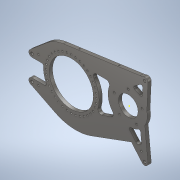
# Autodesk Inventor part: DTR-6
Saved by Autodesk Inventor 2021 (Build 250183000, 183)
## iProperties
Created: 2018-12-06
Part Number: DTR-6
Material: Aluminum 6061
Document SubType Name: Modeling
Designer: Lucas Foulk
Density: 2.7 g/cm^3
Appearance: Semi-Polished
Description: Right Mounting Plate
Material_Size: 1/2 Aluminum Plate
Quantity: 1
Author: Lucas Foulk
Autodesk Inventor part; units mm, degrees
ref_plane "YZ Plane" through (0, 0, 0) normal (1, 0, 0) x (0, 1, 0)
ref_plane "XZ Plane" through (0, 0, 0) normal (0, 1, 0) x (-1, 0, 0)
ref_plane "XY Plane" through (0, 0, 0) normal (0, 0, 1) x (1, 0, 0)
sketch "Sketch14" plane through (0, 0, 0) normal (0, 0, 1) x (1, 0, 0)
  circle A0 centre (0, 0) radius 69.85
  circle A1 centre (59.6616, 114.3) radius 12.7
  circle A2 centre (59.6616, -157.9372) radius 12.7
  circle A3 centre (-225.4026, -38.1) radius 107.95
  line L0 (52.1743, 124.5582) -> (-41.1802, 56.42)
  line L1 (72.3489, 113.732) -> (67.9766, 16.0689)
  line L2 (59.6616, 114.3) -> (0, 0)
  line L3 (0, 0) -> (59.6616, -157.9372)
  line L4 (72.2989, -156.6771) -> (60.2073, -35.4133)
  line L5 (50.0015, -166.1818) -> (-53.1301, -45.3456)
  line L6 (-547.6025, 1708.7209) -> (-492.7385, 1708.7209)
  circle A4 centre (-377.8026, -107.1372) radius 12.7
  circle A5 centre (-377.8026, -12.7) radius 12.7
  line L7 (-377.8026, -25.4) -> (-332.603, -25.4)
  line L8 (-377.8026, -94.4372) -> (-317.4859, -94.4372)
  line L9 (59.6616, 114.3) -> (59.6616, -157.9372)
  line L10 (-380.0803, -119.6313) -> (-244.7629, -144.2997)
  line L11 (-383.8817, -1.5494) -> (-277.0748, 56.6797)
  point P0 (49.5036, 49.279)
  point P1 (31.1227, 62.5332)
  point P2 (49.5036, 49.279)
  point P3 (-216.3804, 69.4723)
  point P4 (27.7497, 64.1013)
  point P5 (-222.5423, 69.8121)
  point P6 (64.0721, 27.817)
  point P7 (-119.2874, -57.9179)
  point P8 (35.0174, 60.4384)
  point P9 (30.2851, 62.9431)
  point P10 (30.2566, 62.9568)
  point P11 (-183.3373, 61.3169)
  point P12 (-197.0061, 66.0482)
  point P13 (-176.345, 58.059)
  dimension "d96" = 215.9
  dimension "d99" = 139.7
  dimension "d97" = 54.864
  dimension "d98" = 228.6
  dimension "d100" = 25.4
  dimension "d101" = 25.4
  dimension "d102" = 152.4
  dimension "d103" = 152.4
  dimension "d104" = 94.4372
  dimension "d105" = 25.4
  dimension "d108" = 272.2372
  dimension "d109" = 38.1
  dimension "d132" = 127
  dimension "d133" = 437.4642
  dimension "d207" = 25
  dimension "d208" = 15
  constraints: 24 end point, 8 point on circle, 8 tangent, 4 centre point, 3 horizontal, 2 coincident, 2 equal radius, 1 vertical, 30 other
  measures "d97" distance of L6.start L6.end
  measures "d98" distance of point (-225.403, -38.1) point (0, 0)
  measures "d100" diameter of A1
  measures "d101" diameter of A4
  measures "d102" horizontal distance of A4.centre point (-225.403, -38.1)
  measures "d103" horizontal distance of A5.centre point (-225.403, -38.1)
  measures "d104" distance of A4.centre A5.centre
  measures "d105" vertical distance of A5.centre point (-225.403, -38.1)
  measures "d108" distance of L9.start L9.end
  measures "d109" vertical distance of point (-225.403, -38.1) point (0, 0)
  measures "d132" vertical distance of L9.start A5.centre
  measures "d133" horizontal distance of L9.start A5.centre
  measures "d207" angle of L2 L1
  measures "d208" angle of L3 L4
extrude "Extrusion13" add sketch "Sketch14" along normal blind 12.7
sketch "Sketch15" plane through (0, 0, 12.7) normal (0, 0, 1) x (1, 0, 0)
  arc A0 (-383.8817, -1.5494) -> (-377.8026, -25.4) centre (-377.8026, -12.7) ccw projected
  arc A1 (-377.8026, -94.4372) -> (-380.0803, -119.6313) centre (-377.8026, -107.1372) ccw projected
  arc A2 (50.0015, -166.1818) -> (72.2989, -156.6771) centre (59.6616, -157.9372) ccw projected
  arc A3 (72.3489, 113.732) -> (52.1743, 124.5582) centre (59.6616, 114.3) ccw projected
  point P0 (0, 0)
  constraints: 4 coincident
hole "Hole4" at (-377.8026, -12.7, 12.7) at (-377.8026, -107.1372, 12.7) at (59.6616, -157.9372, 12.7) at (59.6616, 114.3, 12.7) direction (0, 0, -1) diameter 9.8044 depth 12.2936 tip angle 118 clearance for "Flat Head Machine Screw (82)" size "3/8" standard "Ansi Unified Screw Threads"
sketch "Sketch18" plane through (0, 0, 12.7) normal (0, 0, 1) x (1, 0, 0)
  arc A0 (-244.7629, -144.2997) -> (-277.0748, 56.6797) centre (-225.4026, -38.1) ccw projected
  arc A1 (-41.1802, 56.42) -> (-53.1301, -45.3456) centre (0, 0) ccw projected
  arc A2 (-36.2787, -59.6899) -> (-53.8815, 44.45) centre (0, 0) ccw
  line L0 (-189.9226, -140.0528) -> (22.9577, -65.9694)
  line L1 (-132.5746, -93.2013) -> (-36.2787, -59.6899)
  line L2 (-225.4026, 69.85) -> (0, 69.85)
  line L3 (-155.8419, 44.45) -> (-53.8815, 44.45)
  arc A3 (-155.8419, 44.45) -> (-225.4026, 69.85) centre (-225.4026, -38.1) ccw
  arc A4 (-189.9226, -140.0528) -> (-132.5746, -93.2013) centre (-225.4026, -38.1) ccw
  dimension "d134" = 25.4
  dimension "d135" = 25.4
  constraints: 11 point on circle, 8 end point, 4 tangent, 3 centre point, 2 coincident, 2 parallel, 1 concentric
  measures "d134" distance between parallel lines of L2 L3
  measures "d135" distance between parallel lines of L0 L1
extrude "Extrusion15" add sketch "Sketch18" against normal up to surface (12.7 mm away) contours A0 L1 A2 L0 | A0 L2 A2 A1 L3
sketch "Sketch21" plane through (0, 0, 12.7) normal (0, 0, 1) x (1, 0, 0)
  line L0 (-13.2861, -92.0295) -> (-65.0964, -110.0597)
  line L1 (-0.0132, -107.5811) -> (-71.1332, -132.3311)
  line L2 (-189.9226, -140.0528) -> (-22.1348, -81.6618) projected
  line L3 (-22.1348, -81.6618) -> (50.0015, -166.1818) projected
  line L4 (-65.0964, -110.0597) -> (-73.9451, -99.6921)
  line L5 (-71.1332, -132.3311) -> (-93.2548, -106.4119)
  point P0 (0, 0)
  point P1 (-525.367, -226.8446)
  dimension "d247" = 19.05
  dimension "d249" = 19.05
  dimension "d250" = 12.7
  dimension "d251" = 71.12
  constraints: 8 end point, 4 parallel, 4 point on line
  measures "d247" distance between parallel lines of L1 L0
  measures "d249" distance between parallel lines of L5 L4
  measures "d250" distance between parallel lines of L2 L0
  measures "d251" horizontal distance of L1.start L1.end
extrude "Extrusion17" add sketch "Sketch21" against normal up to surface (12.7 mm away)
sketch "Sketch27" plane through (0, 0, 12.7) normal (0, 0, 1) x (1, 0, 0)
  line L0 (-225.4026, -136.525) -> (-225.4026, 60.325)
  line L1 (-323.8276, -38.1) -> (-126.9776, -38.1)
  circle A0 centre (-225.4026, -38.1) radius 85.725 projected
  point P0 (0, 0)
  point P1 (-300.8006, -101.3664)
  point P2 (-288.669, 37.2979)
  point P3 (-150.0047, 25.1664)
  point P4 (-162.1363, -113.4979)
  point P5 (-242.494, -135.0297)
  point P6 (-322.3323, -21.0087)
  point P7 (-208.3113, 58.8297)
  point P8 (-128.4729, -55.1913)
  point P9 (-176.1901, -123.3386)
  point P10 (-310.6412, -87.3125)
  point P11 (-274.6151, 47.1386)
  point P12 (-140.1641, 11.1125)
  point P13 (-132.9134, -71.7633)
  point P14 (-259.066, -130.5892)
  point P15 (-317.8919, -4.4367)
  point P16 (-191.7393, 54.3892)
  point P17 (-132.9134, -4.4367)
  point P18 (-191.7393, -130.5892)
  point P19 (-317.8919, -71.7633)
  point P20 (-259.066, 54.3892)
  point P21 (-176.1901, 47.1386)
  point P22 (-140.1641, -87.3125)
  point P23 (-274.6151, -123.3386)
  point P24 (-310.6412, 11.1125)
  point P25 (-242.494, 58.8297)
  point P26 (-128.4729, -21.0087)
  point P27 (-208.3113, -135.0297)
  point P28 (-322.3323, -55.1913)
  point P29 (-300.8006, 25.1664)
  point P30 (-162.1363, 37.2979)
  point P31 (-150.0047, -101.3664)
  point P32 (-288.669, -113.4979)
  dimension "d178" = 196.85
  dimension "d181" = 360
  constraints: 5 coincident, 4 end point, 2 midpoint, 1 horizontal, 1 perpendicular, 1 vertical, 37 other
  measures "d178" distance of L0.start L0.end
hole "Hole9" at (-323.8276, -38.1, 12.7) at (-225.4026, -136.525, 12.7) at (-225.4026, 60.325, 12.7) at (-126.9776, -38.1, 12.7) at (-300.8006, -101.3664, 12.7) at (-288.669, 37.2979, 12.7) at (-150.0047, 25.1664, 12.7) at (-162.1363, -113.4979, 12.7) at (-242.494, -135.0297, 12.7) at (-322.3323, -21.0087, 12.7) at (-208.3113, 58.8297, 12.7) at (-128.4729, -55.1913, 12.7) at (-176.1901, -123.3386, 12.7) at (-310.6412, -87.3125, 12.7) at (-274.6151, 47.1386, 12.7) at (-140.1641, 11.1125, 12.7) at (-132.9134, -71.7633, 12.7) at (-259.066, -130.5892, 12.7) at (-317.8919, -4.4367, 12.7) at (-191.7393, 54.3892, 12.7) at (-132.9134, -4.4367, 12.7) at (-191.7393, -130.5892, 12.7) at (-317.8919, -71.7633, 12.7) at (-259.066, 54.3892, 12.7) at (-176.1901, 47.1386, 12.7) at (-140.1641, -87.3125, 12.7) at (-274.6151, -123.3386, 12.7) at (-310.6412, 11.1125, 12.7) at (-242.494, 58.8297, 12.7) at (-128.4729, -21.0087, 12.7) at (-208.3113, -135.0297, 12.7) at (-322.3323, -55.1913, 12.7) at (-300.8006, 25.1664, 12.7) at (-162.1363, 37.2979, 12.7) at (-150.0047, -101.3664, 12.7) at (-288.669, -113.4979, 12.7) direction (0, 0, -1) diameter 6.5278 end through all clearance for "Socket Head Cap Screw" size "1/4" standard "Ansi Unified Screw Threads"
sketch "Sketch29" plane through (0, 0, 12.7) normal (0, 0, 1) x (1, 0, 0)
  circle A0 centre (-377.8026, -12.7) radius 4.9022 projected
  circle A1 centre (-377.8026, -107.1372) radius 4.9022 projected
  circle A2 centre (59.6616, -157.9372) radius 4.9022 projected
  circle A3 centre (59.6616, 114.3) radius 4.9022 projected
  line L0 (-377.8026, -12.7) -> (-352.4026, -2.6443)
  line L1 (-377.8026, -107.1372) -> (-352.4026, -107.1372)
  line L2 (59.6616, -157.9372) -> (46.9616, -128.1441)
  circle A4 centre (59.6616, 114.3) radius 4.9022 projected
  line L3 (-277.0748, 56.6797) -> (-383.8817, -1.5494) projected
  line L4 (52.1743, 124.5582) -> (-22.7801, 69.85) projected
  line L5 (67.9766, 16.0689) -> (72.3489, 113.732) projected
  line L6 (72.2989, -156.6771) -> (60.2073, -35.4133) projected
  line L7 (-53.1301, -45.3456) -> (50.0015, -166.1818) projected
  point P0 (0, 0)
  point P1 (20.7198, 101.6)
  point P2 (22.4341, -133.8818)
  dimension "d191" = 25.4
  dimension "d192" = 7
  dimension "d193" = 25.4
  dimension "d194" = 51.311
  dimension "d197" = 34.786
  dimension "d198" = 17.393
  dimension "d199" = 12.7
  constraints: 6 end point, 3 coincident, 1 horizontal
  measures "d191" distance of L1.start L1.end
  measures "d192" angle of L3 L0
  measures "d193" horizontal distance of L0.start L0.end
  measures "d194" angle of L4 L5
  measures "d197" angle of L6 L7
  measures "d198" angle of L6 L2
  measures "d199" horizontal distance of L2.start L2.end
hole "Hole10" at (-352.4026, -2.6443, 12.7) at (-352.4026, -107.1372, 12.7) at (46.9616, -128.1441, 12.7) direction (0, 0, -1) diameter 6.7564 end through all clearance for "Flat Head Machine Screw (82)" size "1/4" standard "Ansi Unified Screw Threads"
sketch "Sketch31" plane through (0, 0, 12.7) normal (0, 0, 1) x (1, 0, 0)
  circle A0 centre (-352.4026, -107.1372) radius 3.3782 projected
  circle A1 centre (-352.4026, -2.6443) radius 3.3782 projected
  circle A2 centre (46.9616, -128.1441) radius 3.3782 projected
  circle A3 centre (-150.0047, -101.3664) radius 3.2639 projected
  circle A4 centre (-300.8006, 25.1664) radius 3.2639 projected
  circle A5 centre (-208.3113, -135.0297) radius 3.2639 projected
  circle A6 centre (-242.494, 58.8297) radius 3.2639 projected
  circle A7 centre (-274.6151, -123.3386) radius 3.2639 projected
  circle A8 centre (-176.1901, 47.1386) radius 3.2639 projected
  circle A9 centre (-317.8919, -71.7633) radius 3.2639 projected
  circle A10 centre (-132.9134, -4.4367) radius 3.2639 projected
  circle A11 centre (-317.8919, -4.4367) radius 3.2639 projected
  circle A12 centre (-132.9134, -71.7633) radius 3.2639 projected
  circle A13 centre (-274.6151, 47.1386) radius 3.2639 projected
  circle A14 centre (-176.1901, -123.3386) radius 3.2639 projected
  circle A15 centre (-208.3113, 58.8297) radius 3.2639 projected
  circle A16 centre (-242.494, -135.0297) radius 3.2639 projected
  circle A17 centre (-150.0047, 25.1664) radius 3.2639 projected
  circle A18 centre (-300.8006, -101.3664) radius 3.2639 projected
  circle A19 centre (-225.4026, 60.325) radius 3.2639 projected
  circle A20 centre (-323.8276, -38.1) radius 3.2639 projected
  circle A21 centre (-225.4026, -136.525) radius 3.2639 projected
  circle A22 centre (-126.9776, -38.1) radius 3.2639 projected
  circle A23 centre (-288.669, 37.2979) radius 3.2639 projected
  circle A24 centre (-162.1363, -113.4979) radius 3.2639 projected
  circle A25 centre (-322.3323, -21.0087) radius 3.2639 projected
  circle A26 centre (-128.4729, -55.1913) radius 3.2639 projected
  circle A27 centre (-310.6412, -87.3125) radius 3.2639 projected
  circle A28 centre (-140.1641, 11.1125) radius 3.2639 projected
  circle A29 centre (-259.066, -130.5892) radius 3.2639 projected
  circle A30 centre (-191.7393, 54.3892) radius 3.2639 projected
  circle A31 centre (-191.7393, -130.5892) radius 3.2639 projected
  circle A32 centre (-259.066, 54.3892) radius 3.2639 projected
  circle A33 centre (-140.1641, -87.3125) radius 3.2639 projected
  circle A34 centre (-310.6412, 11.1125) radius 3.2639 projected
  circle A35 centre (-128.4729, -21.0087) radius 3.2639 projected
  circle A36 centre (-322.3323, -55.1913) radius 3.2639 projected
  circle A37 centre (-162.1363, 37.2979) radius 3.2639 projected
  circle A38 centre (-288.669, -113.4979) radius 3.2639 projected
  line L0 (-53.8815, 44.45) -> (-155.8419, 44.45) projected
  arc A39 (-132.5746, -93.2013) -> (-155.8419, 44.45) centre (-225.4026, -38.1) ccw projected
  line L1 (-132.5746, -93.2013) -> (-39.832, -60.9264) projected
  arc A40 (-53.8815, 44.45) -> (-53.1301, -45.3456) centre (0, 0) ccw projected
  circle A41 centre (-377.8026, -12.7) radius 4.9022 projected
  circle A42 centre (-377.8026, -107.1372) radius 4.9022 projected
  circle A43 centre (59.6616, -157.9372) radius 4.9022 projected
  circle A44 centre (59.6616, 114.3) radius 4.9022 projected
  arc A45 (60.2073, -35.4133) -> (67.9766, 16.0689) centre (0, 0) ccw projected
  line L2 (60.2073, -35.4133) -> (72.2989, -156.6771) projected
  arc A46 (50.0015, -166.1818) -> (72.2989, -156.6771) centre (59.6616, -157.9372) ccw projected
  line L3 (50.0015, -166.1818) -> (-0.0132, -107.5811) projected
  arc A47 (-244.7629, -144.2997) -> (-189.9226, -140.0528) centre (-225.4026, -38.1) ccw projected
  line L4 (-244.7629, -144.2997) -> (-380.0803, -119.6313) projected
  arc A48 (-377.8026, -94.4372) -> (-380.0803, -119.6313) centre (-377.8026, -107.1372) ccw projected
  line L5 (-377.8026, -94.4372) -> (-317.4859, -94.4372) projected
  arc A49 (-332.603, -25.4) -> (-317.4859, -94.4372) centre (-225.4026, -38.1) ccw projected
  line L6 (-332.603, -25.4) -> (-377.8026, -25.4) projected
  arc A50 (-383.8817, -1.5494) -> (-377.8026, -25.4) centre (-377.8026, -12.7) ccw projected
  line L7 (-383.8817, -1.5494) -> (-277.0748, 56.6797) projected
  arc A51 (-225.4026, 69.85) -> (-277.0748, 56.6797) centre (-225.4026, -38.1) ccw projected
  line L8 (-225.4026, 69.85) -> (-22.7801, 69.85) projected
  line L9 (-22.7801, 69.85) -> (52.1743, 124.5582) projected
  arc A52 (72.3489, 113.732) -> (52.1743, 124.5582) centre (59.6616, 114.3) ccw projected
  line L10 (72.3489, 113.732) -> (67.9766, 16.0689) projected
  circle A53 centre (0, 0) radius 69.85
  arc A54 (60.2073, -35.4133) -> (67.9766, 16.0689) centre (0, 0) ccw projected
  line L11 (8.7745, 69.2967) -> (42.0481, 93.5826)
  line L12 (50.3553, 48.4083) -> (52.1354, 88.1695)
  line L13 (-7.5172, -69.4443) -> (25.0114, -107.5572)
  line L14 (43.019, -55.0308) -> (47.3088, -98.0524)
  arc A55 (52.1354, 88.1695) -> (42.0481, 93.5826) centre (45.7917, 88.4535) ccw
  arc A56 (25.0114, -107.5572) -> (47.3088, -98.0524) centre (34.6715, -99.3125) ccw
  line L15 (-93.2548, -106.4119) -> (-189.9226, -140.0528) projected
  line L16 (-39.832, -60.9264) -> (-53.1301, -45.3456) projected
  line L17 (-0.0132, -107.5811) -> (-71.1332, -132.3311) projected
  line L18 (-71.1332, -132.3311) -> (-93.2548, -106.4119) projected
  point P0 (-3.4437, -126.5534)
  dimension "d210" = 19.05
  dimension "d211" = 19.05
  dimension "d212" = 19.05
  dimension "d213" = 6.35
  dimension "d214" = 12.7
  dimension "d223" = 19.05
  constraints: 8 end point, 8 point on circle, 4 parallel, 4 tangent, 3 centre point, 1 coincident, 1 concentric
  measures "d210" distance between parallel lines of L2 L14
  measures "d211" distance between parallel lines of L9 L11
  measures "d212" distance between parallel lines of L10 L12
  measures "d213" radius of A55
  measures "d214" radius of A56
  measures "d223" distance between parallel lines of L13 L3
extrude "Extrusion18" cut sketch "Sketch31" against normal blind 25.4 contours L11 A55 L12 A53 | A53 L14 A56 L13
sketch "Sketch32" plane through (0, 0, 12.7) normal (0, 0, 1) x (1, 0, 0)
  line L0 (-377.8026, -25.4) -> (-332.603, -25.4) projected
  arc A0 (-333.1859, -32.1028) -> (-339.5261, -25.4) centre (-339.5261, -31.75) ccw
  line L1 (-317.4859, -94.4372) -> (-377.8026, -94.4372) projected
  arc A1 (-328.1926, -94.4372) -> (-322.482, -85.3101) centre (-328.1926, -88.0872) ccw
  line L2 (8.7745, 69.2967) -> (42.0481, 93.5826) projected
  arc A2 (50.3553, 48.4083) -> (8.7745, 69.2967) centre (0, 0) ccw projected
  arc A3 (20.0429, 77.5213) -> (21.8044, 66.3596) centre (23.7866, 72.3923) ccw
  line L3 (52.1354, 88.1695) -> (50.3553, 48.4083) projected
  arc A4 (40.8813, 56.6369) -> (50.9415, 61.5017) centre (44.5978, 61.7857) ccw
  arc A5 (-7.5172, -69.4443) -> (43.019, -55.0308) centre (0, 0) ccw projected
  line L4 (-7.5172, -69.4443) -> (25.0114, -107.5572) projected
  arc A6 (5.8386, -69.6056) -> (1.5394, -80.0557) centre (6.3694, -75.9333) ccw
  arc A7 (-332.603, -25.4) -> (-317.4859, -94.4372) centre (-225.4026, -38.1) ccw projected
  line L5 (43.019, -55.0308) -> (47.3088, -98.0524) projected
  arc A8 (50.3553, 48.4083) -> (40.8813, 56.6369) centre (0, 0) ccw
  arc A9 (21.8044, 66.3596) -> (8.7745, 69.2967) centre (0, 0) ccw
  arc A10 (-7.5172, -69.4443) -> (5.8386, -69.6056) centre (0, 0) ccw
  arc A11 (-322.482, -85.3101) -> (-317.4859, -94.4372) centre (-225.4026, -38.1) ccw
  arc A12 (-332.603, -25.4) -> (-333.1859, -32.1028) centre (-225.4026, -38.1) ccw
  line L6 (-339.5261, -25.4) -> (-332.603, -25.4)
  line L7 (-328.1926, -94.4372) -> (-317.4859, -94.4372)
  line L8 (1.5394, -80.0557) -> (-7.5172, -69.4443)
  line L9 (47.3088, -98.0524) -> (43.019, -55.0308) projected
  line L10 (20.0429, 77.5213) -> (8.7745, 69.2967)
  line L11 (50.9415, 61.5017) -> (50.3553, 48.4083)
  arc A13 (34.6045, -60.6758) -> (43.019, -55.0308) centre (0, 0) ccw
  line L12 (43.019, -55.0308) -> (44.069, -65.5617)
  arc A14 (44.069, -65.5617) -> (34.6045, -60.6758) centre (37.7504, -66.1918) ccw
  dimension "d217" = 6.35
  constraints: 30 point on circle, 15 tangent, 12 centre point, 12 end point, 11 equal radius, 6 point on line, 5 collinear
  measures "d217" radius of A0
extrude "Extrusion19" add sketch "Sketch32" against normal up to surface (12.7 mm away)
sketch "Sketch37" plane through (0, 0, 12.7) normal (0, 0, 1) x (1, 0, 0)
  arc A0 (-132.5746, -93.2013) -> (-155.8419, 44.45) centre (-225.4026, -38.1) ccw projected
  line L0 (-155.8419, 44.45) -> (-53.8815, 44.45) projected
  arc A1 (-53.8815, 44.45) -> (-53.1301, -45.3456) centre (0, 0) ccw projected
  line L1 (-39.832, -60.9264) -> (-132.5746, -93.2013) projected
  line L2 (-53.1301, -45.3456) -> (-39.832, -60.9264) projected
  arc A2 (-121.7328, -68.1961) -> (-105.3623, -83.7313) centre (-109.5364, -71.7368) ccw
  arc A3 (-127.0289, 44.45) -> (-137.384, 24.3974) centre (-127.0289, 31.75) ccw
  arc A4 (-69.5608, 44.45) -> (-51.0868, -64.8432) centre (0, 0) ccw
  line L3 (-127.0289, 44.45) -> (-69.5608, 44.45)
  line L4 (-105.3623, -83.7313) -> (-51.0868, -64.8432)
  arc A5 (-121.7328, -68.1961) -> (-137.384, 24.3974) centre (-225.4026, -38.1) ccw
  point P0 (-64.4769, 26.8654)
  point P1 (-76.2, 44.45)
  point P2 (-57.3797, -67.0331)
  point P3 (-51.8938, -46.794)
  dimension "d305" = 165.1
  constraints: 11 point on circle, 7 point on line, 5 tangent, 4 centre point, 4 end point, 1 coincident, 1 equal radius
  measures "d305" diameter of A4
extrude "Extrusion24" add sketch "Sketch37" against normal up to surface (12.7 mm away) contours A4 L0 A1 L2 L1
fillet "Fillet3" radius 6.35 1 edges at (-71.1332, -132.3311, 6.35)
sketch "Sketch39" plane through (0, 0, 12.7) normal (0, 0, 1) x (1, 0, 0)
  line L0 (-0.0132, -107.5811) -> (50.0015, -166.1818) projected
  line L1 (-67.0339, -130.9046) -> (-0.0132, -107.5811) projected
  arc A0 (5.6223, -114.184) -> (-8.2118, -110.4342) centre (-4.0377, -122.4287) ccw
  line L2 (-93.2548, -106.4119) -> (-73.9509, -129.0297) projected
  line L3 (-189.9226, -140.0528) -> (-93.2548, -106.4119) projected
  arc A1 (-87.6193, -113.0149) -> (-101.4534, -109.2651) centre (-97.2793, -121.2595) ccw
  point P0 (0, 0)
  dimension "d263" = 12.7
  constraints: 4 point on circle, 4 point on line, 4 tangent, 2 centre point, 1 equal radius
  measures "d263" radius of A1
extrude "Extrusion27" add sketch "Sketch39" against normal up to surface (12.7 mm away)
chamfer "Chamfer1" distance 0.3969 angle 45 8 edges at (-377.8026, -7.7978, 12.7) (-377.8026, -102.235, 12.7) (59.6616, 119.2022, 12.7) (59.6616, -153.035, 12.7) (-377.8026, -7.7978, 0.4064) (-377.8026, -102.235, 0.4064) (59.6616, 118.5258, 0) (59.6616, -153.7114, 0)
sketch "Sketch40" plane through (0, 0, 12.7) normal (0, 0, 1) x (1, 0, 0)
  point P0 (0, 0)
sketch "Sketch42" plane through (0, 0, 12.7) normal (0, 0, 1) x (1, 0, 0)
  circle A0 centre (-225.4026, 60.325) radius 3.2639 projected
  circle A1 centre (-225.4026, -136.525) radius 3.2639 projected
  line L0 (-225.4026, 60.325) -> (-225.4026, -136.525)
  circle A2 centre (-4.0416, -1.5494) radius 38.1635
  line L1 (0, 0) -> (-21.5953, 0)
  dimension "d303" = 76.327
  dimension "d304" = 221.361
  dimension "d317" = 1.5494
  constraints: 4 end point, 1 centre point, 1 horizontal, 1 vertical
  measures "d303" diameter of A2
  measures "d304" distance from line of A2.centre L0
  measures "d317" distance from line of A2.centre L1
extrude "Extrusion29" cut sketch "Sketch42" against normal up to surface (12.7 mm away) contours A2
sketch "Sketch43" plane through (0, 0, 12.7) normal (0, 0, 1) x (1, 0, 0)
  circle A0 centre (-225.4026, 60.325) radius 3.2639 projected
  circle A1 centre (-225.4026, -136.525) radius 3.2639 projected
  line L0 (-225.4026, 60.325) -> (-225.4026, -136.525)
  circle A2 centre (-323.8276, -38.1) radius 3.2639 projected
  circle A3 centre (-126.9776, -38.1) radius 3.2639 projected
  line L1 (-323.8276, -38.1) -> (-126.9776, -38.1)
  circle A4 centre (-225.4026, -38.1) radius 85.725
  point P0 (0, 0)
  dimension "d296" = 171.45
  constraints: 4 end point, 1 centre point, 1 horizontal, 1 midpoint, 1 vertical
  measures "d296" diameter of A4
extrude "Extrusion30" cut sketch "Sketch43" against normal blind 25.4 contours A4 L1 L0 | L0 L1 A4 | L1 A4 L0 | L0 A4 L1
fillet "Fillet4" radius 12.7 2 edges at (-69.5608, 44.45, 6.35) (-51.0868, -64.8432, 6.35)
fillet "Fillet5" radius 12.7 2 edges at (-155.8419, 44.45, 6.35) (-132.5746, -93.2013, 6.35)
sketch "Sketch45" plane through (0, 0, 12.7) normal (0, 0, 1) x (1, 0, 0)
  circle A0 centre (-4.0416, -1.5494) radius 38.1635 projected
  circle A1 centre (-4.0416, -1.5494) radius 56.388
  circle A2 centre (-4.0416, 54.8386) radius 4.1275
  circle A3 centre (49.5865, 15.8755) radius 4.1275
  circle A4 centre (29.1024, -47.1683) radius 4.1275
  circle A5 centre (-37.1857, -47.1683) radius 4.1275
  circle A6 centre (-57.6698, 15.8755) radius 4.1275
  point P0 (0, 0)
  dimension "d308" = 112.776
  dimension "d309" = 8.255
  dimension "d312" = 360
  constraints: 5 centre point, 1 coincident, 1 vertical alignment, 13 other
  measures "d309" diameter of A2
extrude "Extrusion32" cut sketch "Sketch45" against normal blind 25.4 contours A3 A1 | A1 A3 | A4 A1 | A1 A4 | A2 A1 | A1 A2 | A5 A1 | A1 A5 | A6 A1 | A1 A6
sketch "Sketch48" plane through (0, 0, 12.7) normal (0, 0, 1) x (1, 0, 0)
  line L0 (-277.0748, 56.6797) -> (-383.8817, -1.5494) projected
  line L1 (-383.8817, -1.5494) -> (-292.1, 76.1736)
  arc A0 (72.3489, 113.732) -> (52.1743, 124.5582) centre (59.6616, 114.3) ccw projected
  arc A1 (-225.4026, 69.85) -> (-277.0748, 56.6797) centre (-225.4026, -38.1) ccw projected
  line L2 (-383.8817, -1.5494) -> (-277.0748, 56.6797)
  arc A2 (-277.0748, 56.6797) -> (-225.4026, 69.85) centre (-225.4026, -38.1) ccw
  line L3 (52.1743, 124.5582) -> (-22.7801, 69.85) projected
  line L4 (-22.7801, 69.85) -> (-225.4026, 69.85) projected
  arc A3 (-225.4026, 69.85) -> (-277.0748, 56.6797) centre (-225.4026, -38.1) ccw
  line L5 (-225.4026, 69.85) -> (-22.7801, 69.85)
  line L6 (52.1743, 124.5582) -> (-22.7801, 69.85)
  line L7 (-292.1, 76.1736) -> (52.1743, 124.5582)
  point P0 (0, 0)
  dimension "d332" = 8
  dimension "d335" = 292.1
  constraints: 10 end point, 5 point on circle, 5 tangent, 3 collinear, 2 centre point
  measures "d332" angle of L7 L4
  measures "d335" horizontal distance of L1.end point (0, 0)
extrude "Extrusion35" add sketch "Sketch48" against normal blind 12.7 contours L0 L1 L7 L3 L4 A1
fillet "Fillet6" radius 127 1 edges at (-292.1, 76.1736, 6.35)
fillet "Fillet7" radius 76.2 1 edges at (52.1743, 124.5582, 6.35)
sketch "Sketch49" plane through (0, 0, 12.7) normal (0, 0, 1) x (1, 0, 0)
  line L0 (-380.0803, -119.6313) -> (-244.7629, -144.2997) projected
  arc A0 (-244.7629, -144.2997) -> (-189.9226, -140.0528) centre (-225.4026, -38.1) ccw projected
  line L1 (-189.9226, -140.0528) -> (-101.4534, -109.2651) projected
  line L2 (-87.6193, -113.0149) -> (-73.9509, -129.0297) projected
  arc A1 (-87.6193, -113.0149) -> (-101.4534, -109.2651) centre (-97.2793, -121.2595) ccw projected
  line L3 (-244.7629, -144.2997) -> (-380.0803, -119.6313)
  arc A2 (-244.7629, -144.2997) -> (-189.9226, -140.0528) centre (-225.4026, -38.1) ccw
  line L4 (-189.9226, -140.0528) -> (-101.4534, -109.2651)
  arc A3 (-87.6193, -113.0149) -> (-101.4534, -109.2651) centre (-97.2793, -121.2595) ccw
  line L5 (-87.6193, -113.0149) -> (-73.9509, -129.0297)
  line L6 (-380.0803, -119.6313) -> (-219.0526, -200.66)
  arc A4 (-73.9509, -129.0297) -> (-67.0339, -130.9046) centre (-69.1209, -124.9073) ccw projected
  arc A5 (5.6223, -114.184) -> (-8.2118, -110.4342) centre (-4.0377, -122.4287) ccw projected
  arc A6 (5.6223, -114.184) -> (-8.2118, -110.4342) centre (-4.0377, -122.4287) ccw
  line L7 (5.6223, -114.184) -> (50.0015, -166.1818) projected
  line L8 (-219.0526, -200.66) -> (8.1328, -117.1254)
  line L9 (8.1328, -117.1254) -> (5.6223, -114.184)
  line L10 (-8.2118, -110.4342) -> (-67.0339, -130.9046) projected
  line L11 (-8.2118, -110.4342) -> (-67.0339, -130.9046)
  arc A7 (-73.9509, -129.0297) -> (-67.0339, -130.9046) centre (-69.1209, -124.9073) ccw
  point P0 (0, 0)
  dimension "d381" = 162.56
  dimension "d382" = 6.35
  dimension "d383" = 1
  constraints: 14 end point, 8 point on circle, 6 tangent, 4 centre point, 3 collinear, 3 point on line, 2 coincident
  measures "d381" vertical distance of L6.end A0.centre
  measures "d382" horizontal distance of L6.end A0.centre
  measures "d383" angle of L8 L10
extrude "Extrusion36" add sketch "Sketch49" against normal blind 12.7
fillet "Fillet8" radius 177.8 1 edges at (-219.0526, -200.66, 6.35)
sketch "Sketch51" plane through (-255.7302, 81.285, 12.7) normal (-0.1391731, 0.9902681, 0) x (0.9902681, 0.1391731, 0)
  line L0 (13.2462, 12.7) -> (13.2462, 0) projected
  line L1 (159.3788, 0) -> (159.3788, 12.7) projected
  line L2 (0, 0) -> (0, 12.7) projected
  point P0 (241.9288, 12.7)
  point P1 (57.15, 6.35)
  point P2 (212.725, 6.35)
  dimension "d353" = 57.15
  dimension "d354" = 212.725
  dimension "d355" = 6.35
  constraints: 1 horizontal alignment
  measures "d353" distance from line of point (57.15, 6.35) L2
  measures "d354" distance from line of point (212.725, 6.35) L2
  measures "d355" vertical distance of point (57.15, 6.35) L2.start
hole "Hole12" at (-199.1364, 89.2388, 6.35) at (-45.0754, 110.8906, 6.35) direction (0.1391731, -0.9902681, 0) diameter 4.9784 depth 16.51 tip angle 118 thread size "1/4-20 UNC" class "1B" standard "ANSI Unified Screw Threads"
sketch "Sketch54" plane through (-380.0803, -119.6313, 0) normal (-0.4494971, -0.8932818, 0) x (0.8932818, -0.4494971, 0)
  line L0 (103.1409, 0) -> (0, 0) projected
  point P0 (285.7449, 0)
  point P1 (44.45, 6.35)
  dimension "d370" = 6.35
  dimension "d371" = 44.45
  measures "d370" distance from line of point (44.45, 6.35) L0
  measures "d371" horizontal distance of point (44.45, 6.35) L0.end
hole "Hole14" at (-340.3739, -139.6114, 6.35) direction (0.4494971, 0.8932818, 0) diameter 4.9784 depth 16.51 tip angle 118 thread size "1/4-20 UNC" class "1B" standard "ANSI Unified Screw Threads"
fillet "Fillet9" radius 76.2 1 edges at (-380.0803, -119.6313, 6.35)
body "Solid2"
